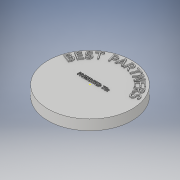
# Autodesk Inventor part: BEST PARTNERS
Saved by Autodesk Inventor 2018.2 (Build 222227000, 227)
## iProperties
Created: 2018-03-07
Part Number: BEST PARTNERS
Material: Generic
Document SubType Name: Modeling
Designer: battin.michael
Density: 1 g/cm^3
Appearance: Default
Author: battin.michael
Autodesk Inventor part; units mm, degrees
ref_plane "YZ Plane" through (0, 0, 0) normal (1, 0, 0) x (0, 1, 0)
ref_plane "XZ Plane" through (0, 0, 0) normal (0, 1, 0) x (-1, 0, 0)
ref_plane "XY Plane" through (0, 0, 0) normal (0, 0, 1) x (1, 0, 0)
sketch "Sketch1" plane through (0, 0, 0) normal (0, 1, 0) x (-1, 0, 0)
  circle A0 centre (0, 0) radius 104.775
  dimension "d0" = 209.55
  constraints: 1 centre point, 1 coincident
  measures "d0" diameter of A0
extrude "Extrusion1" add sketch "Sketch1" along normal blind 25.4
sketch "Sketch2" plane through (0, 25.4, 0) normal (0, 1, 0) x (1, 0, 0)
  circle A0 centre (0, 0) radius 104.775
  circle A1 centre (0, 0) radius 104.775 projected
  spline S0 degree 2 poles (-32.6567, 10.8601) (-32.6567, 10.3661) (-33.0087, 9.4769) (-33.3236, 9.1681) knots 0 0 0 1 2 2 2
  spline S1 degree 2 poles (-33.3236, 9.1681) (-33.7188, 8.7791) (-34.7871, 8.3777) (-35.6022, 8.3777) knots 0 0 0 1 2 2 2
  line L0 (-35.6022, 8.3777) -> (-36.4605, 8.3777)
  line L1 (-36.4605, 8.3777) -> (-36.4605, 5.5372)
  line L2 (-36.4605, 5.5372) -> (-37.4732, 5.5372)
  line L3 (-37.4732, 5.5372) -> (-37.4732, 13.1572)
  line L4 (-37.4732, 13.1572) -> (-35.559, 13.1572)
  spline S2 degree 2 poles (-35.559, 13.1572) (-34.8797, 13.1572) (-33.9288, 12.9349) (-33.5644, 12.6817) knots 0 0 0 1 2 2 2
  spline S3 degree 2 poles (-33.5644, 12.6817) (-33.1384, 12.3915) (-32.6567, 11.4961) (-32.6567, 10.8601) knots 0 0 0 1 2 2 2
  spline S4 degree 2 poles (-33.7126, 10.8292) (-33.7126, 11.2244) (-33.9843, 11.8049) (-34.2622, 11.9901) knots 0 0 0 1 2 2 2
  spline S5 degree 2 poles (-34.2622, 11.9901) (-34.503, 12.1507) (-35.1452, 12.2803) (-35.6207, 12.2803) knots 0 0 0 1 2 2 2
  line L5 (-35.6207, 12.2803) -> (-36.4605, 12.2803)
  line L6 (-36.4605, 12.2803) -> (-36.4605, 9.2422)
  line L7 (-36.4605, 9.2422) -> (-35.7689, 9.2422)
  spline S6 degree 2 poles (-35.7689, 9.2422) (-35.1514, 9.2422) (-34.3919, 9.4398) (-34.1449, 9.6992) knots 0 0 0 1 2 2 2
  spline S7 degree 2 poles (-34.1449, 9.6992) (-33.9164, 9.9277) (-33.7126, 10.4649) (-33.7126, 10.8292) knots 0 0 0 1 2 2 2
  line L8 (-25.7962, 5.5372) -> (-27.1115, 5.5372)
  line L9 (-27.1115, 5.5372) -> (-29.5198, 8.5691)
  line L10 (-29.5198, 8.5691) -> (-30.6807, 8.5691)
  line L11 (-30.6807, 8.5691) -> (-30.6807, 5.5372)
  line L12 (-30.6807, 5.5372) -> (-31.6934, 5.5372)
  line L13 (-31.6934, 5.5372) -> (-31.6934, 13.1572)
  line L14 (-31.6934, 13.1572) -> (-29.7297, 13.1572)
  spline S8 degree 2 poles (-29.7297, 13.1572) (-29.0752, 13.1572) (-28.1921, 13.0152) (-27.7908, 12.7558) knots 0 0 0 1 2 2 2
  spline S9 degree 2 poles (-27.7908, 12.7558) (-27.3894, 12.4965) (-26.9263, 11.6875) (-26.9263, 11.0886) knots 0 0 0 1 2 2 2
  spline S10 degree 2 poles (-26.9263, 11.0886) (-26.9263, 10.2549) (-27.7784, 9.1249) (-28.5071, 8.8532) knots 0 0 0 1 2 2 2
  line L15 (-28.5071, 8.8532) -> (-25.7962, 5.5372)
  spline S11 degree 2 poles (-27.9822, 11.0083) (-27.9822, 11.3417) (-28.2168, 11.8543) (-28.4638, 12.021) knots 0 0 0 1 2 2 2
  spline S12 degree 2 poles (-28.4638, 12.021) (-28.68, 12.163) (-29.2543, 12.2803) (-29.6742, 12.2803) knots 0 0 0 1 2 2 2
  line L16 (-29.6742, 12.2803) -> (-30.6807, 12.2803)
  line L17 (-30.6807, 12.2803) -> (-30.6807, 9.4151)
  line L18 (-30.6807, 9.4151) -> (-29.7915, 9.4151)
  spline S13 degree 2 poles (-29.7915, 9.4151) (-29.3531, 9.4151) (-28.6553, 9.5695) (-28.4144, 9.8103) knots 0 0 0 1 2 2 2
  spline S14 degree 2 poles (-28.4144, 9.8103) (-28.1921, 10.0203) (-27.9822, 10.6131) (-27.9822, 11.0083) knots 0 0 0 1 2 2 2
  line L19 (-25.1911, 5.5372) -> (-25.1911, 13.1572)
  line L20 (-25.1911, 13.1572) -> (-20.4239, 13.1572)
  line L21 (-20.4239, 13.1572) -> (-20.4239, 12.2556)
  line L22 (-20.4239, 12.2556) -> (-24.1784, 12.2556)
  line L23 (-24.1784, 12.2556) -> (-24.1784, 10.1685)
  line L24 (-24.1784, 10.1685) -> (-20.6771, 10.1685)
  line L25 (-20.6771, 10.1685) -> (-20.6771, 9.2669)
  line L26 (-20.6771, 9.2669) -> (-24.1784, 9.2669)
  line L27 (-24.1784, 9.2669) -> (-24.1784, 6.4388)
  line L28 (-24.1784, 6.4388) -> (-20.4239, 6.4388)
  line L29 (-20.4239, 6.4388) -> (-20.4239, 5.5372)
  line L30 (-20.4239, 5.5372) -> (-25.1911, 5.5372)
  spline S15 degree 2 poles (-17.1882, 5.4013) (-18.0157, 5.4013) (-19.1766, 5.7472) (-19.6891, 5.9942) knots 0 0 0 1 2 2 2
  line L31 (-19.6891, 5.9942) -> (-19.6891, 7.2662)
  line L32 (-19.6891, 7.2662) -> (-19.615, 7.2662)
  spline S16 degree 2 poles (-19.615, 7.2662) (-19.1148, 6.7969) (-17.849, 6.2782) (-17.2623, 6.2782) knots 0 0 0 1 2 2 2
  spline S17 degree 2 poles (-17.2623, 6.2782) (-16.4225, 6.2782) (-15.5642, 6.976) (-15.5642, 7.5503) knots 0 0 0 1 2 2 2
  spline S18 degree 2 poles (-15.5642, 7.5503) (-15.5642, 8.0072) (-16.015, 8.5753) (-16.5028, 8.7173) knots 0 0 0 1 2 2 2
  spline S19 degree 2 poles (-16.5028, 8.7173) (-16.8548, 8.8161) (-17.4414, 8.952) (-17.8798, 9.0631) knots 0 0 0 1 2 2 2
  spline S20 degree 2 poles (-17.8798, 9.0631) (-18.275, 9.1681) (-18.8987, 9.4831) (-19.1395, 9.7362) knots 0 0 0 1 2 2 2
  spline S21 degree 2 poles (-19.1395, 9.7362) (-19.3742, 9.9894) (-19.6335, 10.6687) (-19.6335, 11.1133) knots 0 0 0 1 2 2 2
  spline S22 degree 2 poles (-19.6335, 11.1133) (-19.6335, 12.0395) (-18.1886, 13.2931) (-17.0709, 13.2931) knots 0 0 0 1 2 2 2
  spline S23 degree 2 poles (-17.0709, 13.2931) (-16.4287, 13.2931) (-15.2925, 13.0399) (-14.8047, 12.799) knots 0 0 0 1 2 2 2
  line L33 (-14.8047, 12.799) -> (-14.8047, 11.5887)
  line L34 (-14.8047, 11.5887) -> (-14.8788, 11.5887)
  spline S24 degree 2 poles (-14.8788, 11.5887) (-15.2431, 11.9222) (-16.3793, 12.4162) (-17.003, 12.4162) knots 0 0 0 1 2 2 2
  spline S25 degree 2 poles (-17.003, 12.4162) (-17.7069, 12.4162) (-18.5776, 11.7555) (-18.5776, 11.2182) knots 0 0 0 1 2 2 2
  spline S26 degree 2 poles (-18.5776, 11.2182) (-18.5776, 10.7366) (-18.0651, 10.1623) (-17.5834, 10.0326) knots 0 0 0 1 2 2 2
  spline S27 degree 2 poles (-17.5834, 10.0326) (-17.2623, 9.9462) (-16.3299, 9.7239) (-16.0211, 9.6313) knots 0 0 0 1 2 2 2
  spline S28 degree 2 poles (-16.0211, 9.6313) (-15.2369, 9.3904) (-14.5083, 8.4209) (-14.5083, 7.7108) knots 0 0 0 1 2 2 2
  spline S29 degree 2 poles (-14.5083, 7.7108) (-14.5083, 7.26) (-14.8726, 6.3955) (-15.1999, 6.093) knots 0 0 0 1 2 2 2
  spline S30 degree 2 poles (-15.1999, 6.093) (-15.5642, 5.7595) (-16.4904, 5.4013) (-17.1882, 5.4013) knots 0 0 0 1 2 2 2
  line L35 (-13.477, 5.5372) -> (-13.477, 13.1572)
  line L36 (-13.477, 13.1572) -> (-8.7099, 13.1572)
  line L37 (-8.7099, 13.1572) -> (-8.7099, 12.2556)
  line L38 (-8.7099, 12.2556) -> (-12.4643, 12.2556)
  line L39 (-12.4643, 12.2556) -> (-12.4643, 10.1685)
  line L40 (-12.4643, 10.1685) -> (-8.9631, 10.1685)
  line L41 (-8.9631, 10.1685) -> (-8.9631, 9.2669)
  line L42 (-8.9631, 9.2669) -> (-12.4643, 9.2669)
  line L43 (-12.4643, 9.2669) -> (-12.4643, 6.4388)
  line L44 (-12.4643, 6.4388) -> (-8.7099, 6.4388)
  line L45 (-8.7099, 6.4388) -> (-8.7099, 5.5372)
  line L46 (-8.7099, 5.5372) -> (-13.477, 5.5372)
  line L47 (-2.1458, 5.5372) -> (-3.282, 5.5372)
  line L48 (-3.282, 5.5372) -> (-6.6536, 12.1074)
  line L49 (-6.6536, 12.1074) -> (-6.6536, 5.5372)
  line L50 (-6.6536, 5.5372) -> (-7.5984, 5.5372)
  line L51 (-7.5984, 5.5372) -> (-7.5984, 13.1572)
  line L52 (-7.5984, 13.1572) -> (-6.1596, 13.1572)
  line L53 (-6.1596, 13.1572) -> (-3.0906, 7.1242)
  line L54 (-3.0906, 7.1242) -> (-3.0906, 13.1572)
  line L55 (-3.0906, 13.1572) -> (-2.1458, 13.1572)
  line L56 (-2.1458, 13.1572) -> (-2.1458, 5.5372)
  line L57 (1.1763, 5.5372) -> (1.1763, 12.2556)
  line L58 (1.1763, 12.2556) -> (-1.3801, 12.2556)
  line L59 (-1.3801, 12.2556) -> (-1.3801, 13.1572)
  line L60 (-1.3801, 13.1572) -> (4.7455, 13.1572)
  line L61 (4.7455, 13.1572) -> (4.7455, 12.2556)
  line L62 (4.7455, 12.2556) -> (2.1891, 12.2556)
  line L63 (2.1891, 12.2556) -> (2.1891, 5.5372)
  line L64 (2.1891, 5.5372) -> (1.1763, 5.5372)
  line L65 (5.5174, 5.5372) -> (5.5174, 13.1572)
  line L66 (5.5174, 13.1572) -> (10.2845, 13.1572)
  line L67 (10.2845, 13.1572) -> (10.2845, 12.2556)
  line L68 (10.2845, 12.2556) -> (6.5301, 12.2556)
  line L69 (6.5301, 12.2556) -> (6.5301, 10.1685)
  line L70 (6.5301, 10.1685) -> (10.0314, 10.1685)
  line L71 (10.0314, 10.1685) -> (10.0314, 9.2669)
  line L72 (10.0314, 9.2669) -> (6.5301, 9.2669)
  line L73 (6.5301, 9.2669) -> (6.5301, 6.4388)
  line L74 (6.5301, 6.4388) -> (10.2845, 6.4388)
  line L75 (10.2845, 6.4388) -> (10.2845, 5.5372)
  line L76 (10.2845, 5.5372) -> (5.5174, 5.5372)
  spline S31 degree 2 poles (17.4044, 9.341) (17.4044, 8.2974) (16.5584, 6.6178) (15.8482, 6.1485) knots 0 0 0 1 2 2 2
  spline S32 degree 2 poles (15.8482, 6.1485) (15.2678, 5.7842) (14.076, 5.5372) (13.1498, 5.5372) knots 0 0 0 1 2 2 2
  line L77 (13.1498, 5.5372) -> (11.396, 5.5372)
  line L78 (11.396, 5.5372) -> (11.396, 13.1572)
  line L79 (11.396, 13.1572) -> (13.1312, 13.1572)
  spline S33 degree 2 poles (13.1312, 13.1572) (14.2057, 13.1572) (15.4283, 12.8361) (15.8606, 12.552) knots 0 0 0 1 2 2 2
  spline S34 degree 2 poles (15.8606, 12.552) (16.5954, 12.0642) (17.4044, 10.4525) (17.4044, 9.341) knots 0 0 0 1 2 2 2
  spline S35 degree 2 poles (16.3484, 9.3534) (16.3484, 10.2302) (15.768, 11.4714) (15.1937, 11.8234) knots 0 0 0 1 2 2 2
  spline S36 degree 2 poles (15.1937, 11.8234) (14.7861, 12.0642) (13.8661, 12.2803) (13.1806, 12.2803) knots 0 0 0 1 2 2 2
  line L80 (13.1806, 12.2803) -> (12.4087, 12.2803)
  line L81 (12.4087, 12.2803) -> (12.4087, 6.4141)
  line L82 (12.4087, 6.4141) -> (13.1806, 6.4141)
  spline S37 degree 2 poles (13.1806, 6.4141) (13.8537, 6.4141) (14.8726, 6.6302) (15.2863, 6.9204) knots 0 0 0 1 2 2 2
  spline S38 degree 2 poles (15.2863, 6.9204) (15.8174, 7.2786) (16.3484, 8.4642) (16.3484, 9.3534) knots 0 0 0 1 2 2 2
  line L83 (23.5547, 5.5372) -> (23.5547, 12.2556)
  line L84 (23.5547, 12.2556) -> (20.9982, 12.2556)
  line L85 (20.9982, 12.2556) -> (20.9982, 13.1572)
  line L86 (20.9982, 13.1572) -> (27.1239, 13.1572)
  line L87 (27.1239, 13.1572) -> (27.1239, 12.2556)
  line L88 (27.1239, 12.2556) -> (24.5674, 12.2556)
  line L89 (24.5674, 12.2556) -> (24.5674, 5.5372)
  line L90 (24.5674, 5.5372) -> (23.5547, 5.5372)
  spline S39 degree 2 poles (33.2866, 12.2865) (33.7188, 11.7802) (34.2005, 10.2982) (34.2005, 9.3472) knots 0 0 0 1 2 2 2
  spline S40 degree 2 poles (34.2005, 9.3472) (34.2005, 8.4209) (33.7312, 6.9204) (33.2866, 6.4141) knots 0 0 0 1 2 2 2
  spline S41 degree 2 poles (33.2866, 6.4141) (32.8173, 5.883) (31.5761, 5.3766) (30.8289, 5.3766) knots 0 0 0 1 2 2 2
  spline S42 degree 2 poles (30.8289, 5.3766) (30.057, 5.3766) (28.822, 5.9015) (28.3712, 6.4141) knots 0 0 0 1 2 2 2
  spline S43 degree 2 poles (28.3712, 6.4141) (27.9328, 6.9204) (27.4635, 8.4086) (27.4635, 9.3472) knots 0 0 0 1 2 2 2
  spline S44 degree 2 poles (27.4635, 9.3472) (27.4635, 10.3043) (27.939, 11.7616) (28.3774, 12.2865) knots 0 0 0 1 2 2 2
  spline S45 degree 2 poles (28.3774, 12.2865) (28.822, 12.7929) (30.0632, 13.3178) (30.8289, 13.3178) knots 0 0 0 1 2 2 2
  spline S46 degree 2 poles (30.8289, 13.3178) (31.6069, 13.3178) (32.8543, 12.7743) (33.2866, 12.2865) knots 0 0 0 1 2 2 2
  spline S47 degree 2 poles (33.1445, 9.3472) (33.1445, 10.1006) (32.8173, 11.2676) (32.5209, 11.6505) knots 0 0 0 1 2 2 2
  spline S48 degree 2 poles (32.5209, 11.6505) (32.2183, 12.0457) (31.3661, 12.4409) (30.8351, 12.4409) knots 0 0 0 1 2 2 2
  spline S49 degree 2 poles (30.8351, 12.4409) (30.2855, 12.4409) (29.458, 12.058) (29.1431, 11.6505) knots 0 0 0 1 2 2 2
  spline S50 degree 2 poles (29.1431, 11.6505) (28.8405, 11.2615) (28.5194, 10.0882) (28.5194, 9.3472) knots 0 0 0 1 2 2 2
  spline S51 degree 2 poles (28.5194, 9.3472) (28.5194, 7.8467) (29.7791, 6.2535) (30.8351, 6.2535) knots 0 0 0 1 2 2 2
  spline S52 degree 2 poles (30.8351, 6.2535) (31.891, 6.2535) (33.1445, 7.8467) (33.1445, 9.3472) knots 0 0 0 1 2 2 2
  line L91 (37.0039, 5.5372) -> (35.7813, 5.5372)
  line L92 (35.7813, 5.5372) -> (35.7813, 6.9945)
  line L93 (35.7813, 6.9945) -> (37.0039, 6.9945)
  line L94 (37.0039, 6.9945) -> (37.0039, 5.5372)
  line L95 (37.0039, 9.798) -> (35.7813, 9.798)
  line L96 (35.7813, 9.798) -> (35.7813, 11.2553)
  line L97 (35.7813, 11.2553) -> (37.0039, 11.2553)
  line L98 (37.0039, 11.2553) -> (37.0039, 9.798)
  spline S53 degree 2 poles (-76.2187, 36.9163) (-74.8015, 36.3811) (-73.0366, 34.4825) (-72.6654, 33.3214) knots 0 0 0 1 2 2 2
  spline S54 degree 2 poles (-72.6654, 33.3214) (-72.2408, 31.9289) (-72.4572, 29.2119) (-73.1902, 27.2709) knots 0 0 0 1 2 2 2
  line L99 (-73.1902, 27.2709) -> (-75.2497, 21.8176)
  line L100 (-75.2497, 21.8176) -> (-94.2593, 28.9966)
  line L101 (-94.2593, 28.9966) -> (-92.3569, 34.034)
  spline S55 degree 2 poles (-92.3569, 34.034) (-91.5889, 36.0674) (-90.5591, 38.002) (-89.7017, 38.7343) knots 0 0 0 1 2 2 2
  spline S56 degree 2 poles (-89.7017, 38.7343) (-88.7728, 39.5628) (-86.6463, 39.8334) (-85.4447, 39.3796) knots 0 0 0 1 2 2 2
  spline S57 degree 2 poles (-85.4447, 39.3796) (-84.1045, 38.8735) (-82.5139, 36.6534) (-82.3843, 35.1787) knots 0 0 0 1 2 2 2
  line L102 (-82.3843, 35.1787) -> (-82.2919, 35.1438)
  spline S58 degree 2 poles (-82.2919, 35.1438) (-81.1898, 36.6638) (-78.0365, 37.6028) (-76.2187, 36.9163) knots 0 0 0 1 2 2 2
  spline S59 degree 2 poles (-77.1057, 34.2414) (-78.1841, 34.6486) (-79.8032, 34.556) (-80.6452, 33.8179) knots 0 0 0 1 2 2 2
  spline S60 degree 2 poles (-80.6452, 33.8179) (-81.1802, 33.3334) (-81.9003, 31.986) (-82.3948, 30.6766) knots 0 0 0 1 2 2 2
  line L103 (-82.3948, 30.6766) -> (-83.4769, 27.8113)
  line L104 (-83.4769, 27.8113) -> (-76.4523, 25.1584)
  line L105 (-76.4523, 25.1584) -> (-75.6785, 27.2073)
  spline S61 degree 2 poles (-75.6785, 27.2073) (-75.0502, 28.871) (-74.6369, 30.8976) (-74.8506, 31.8232) knots 0 0 0 1 2 2 2
  spline S62 degree 2 poles (-74.8506, 31.8232) (-75.0914, 32.7238) (-76.1044, 33.8632) (-77.1057, 34.2414) knots 0 0 0 1 2 2 2
  spline S63 degree 2 poles (-86.0853, 36.6116) (-86.7631, 36.8676) (-87.9543, 36.7894) (-88.439, 36.3916) knots 0 0 0 1 2 2 2
  spline S64 degree 2 poles (-88.439, 36.3916) (-89.0106, 35.9034) (-89.729, 34.4673) (-90.2351, 33.1271) knots 0 0 0 1 2 2 2
  line L106 (-90.2351, 33.1271) -> (-91.1485, 30.7085)
  line L107 (-91.1485, 30.7085) -> (-85.5873, 28.6083)
  line L108 (-85.5873, 28.6083) -> (-84.5053, 31.4736)
  spline S65 degree 2 poles (-84.5053, 31.4736) (-84.0573, 32.6598) (-83.8791, 33.8774) (-84.0373, 34.6237) knots 0 0 0 1 2 2 2
  spline S66 degree 2 poles (-84.0373, 34.6237) (-84.1859, 35.3487) (-85.1918, 36.2742) (-86.0853, 36.6116) knots 0 0 0 1 2 2 2
  line L109 (-69.019, 37.0158) -> (-86.1686, 47.915)
  line L110 (-86.1686, 47.915) -> (-79.35, 58.644)
  line L111 (-79.35, 58.644) -> (-77.321, 57.3544)
  line L112 (-77.321, 57.3544) -> (-82.6911, 48.9047)
  line L113 (-82.6911, 48.9047) -> (-77.9937, 45.9194)
  line L114 (-77.9937, 45.9194) -> (-72.9857, 53.7993)
  line L115 (-72.9857, 53.7993) -> (-70.9567, 52.5097)
  line L116 (-70.9567, 52.5097) -> (-75.9647, 44.6298)
  line L117 (-75.9647, 44.6298) -> (-69.5996, 40.5846)
  line L118 (-69.5996, 40.5846) -> (-64.2294, 49.0343)
  line L119 (-64.2294, 49.0343) -> (-62.2004, 47.7448)
  line L120 (-62.2004, 47.7448) -> (-69.019, 37.0158)
  spline S67 degree 2 poles (-56.098, 53.8234) (-57.6268, 52.2323) (-60.4367, 50.6389) (-61.8586, 50.1098) knots 0 0 0 1 2 2 2
  line L121 (-61.8586, 50.1098) -> (-64.3046, 52.4601)
  line L122 (-64.3046, 52.4601) -> (-64.1676, 52.6026)
  spline S68 degree 2 poles (-64.1676, 52.6026) (-62.3411, 52.6972) (-59.0048, 54.173) (-57.9209, 55.301) knots 0 0 0 1 2 2 2
  spline S69 degree 2 poles (-57.9209, 55.301) (-56.3693, 56.9158) (-56.1252, 59.8555) (-57.2294, 60.9165) knots 0 0 0 1 2 2 2
  spline S70 degree 2 poles (-57.2294, 60.9165) (-58.1081, 61.7608) (-60.0333, 61.9437) (-61.2077, 61.2681) knots 0 0 0 1 2 2 2
  spline S71 degree 2 poles (-61.2077, 61.2681) (-62.048, 60.7738) (-63.3931, 59.8968) (-64.4169, 59.2591) knots 0 0 0 1 2 2 2
  spline S72 degree 2 poles (-64.4169, 59.2591) (-65.349, 58.6932) (-67.1068, 58.0758) (-68.0386, 58.0805) knots 0 0 0 1 2 2 2
  spline S73 degree 2 poles (-68.0386, 58.0805) (-68.959, 58.0971) (-70.7443, 58.8534) (-71.5992, 59.6749) knots 0 0 0 1 2 2 2
  spline S74 degree 2 poles (-71.5992, 59.6749) (-73.3803, 61.3862) (-73.1209, 66.4808) (-71.0558, 68.6299) knots 0 0 0 1 2 2 2
  spline S75 degree 2 poles (-71.0558, 68.6299) (-69.8692, 69.8648) (-67.2831, 71.5817) (-65.9187, 72.0748) knots 0 0 0 1 2 2 2
  line L123 (-65.9187, 72.0748) -> (-63.5915, 69.8386)
  line L124 (-63.5915, 69.8386) -> (-63.7284, 69.6961)
  spline S76 degree 2 poles (-63.7284, 69.6961) (-65.0427, 69.6117) (-68.0919, 68.3396) (-69.2442, 67.1404) knots 0 0 0 1 2 2 2
  spline S77 degree 2 poles (-69.2442, 67.1404) (-70.5449, 65.7868) (-70.8831, 62.8918) (-69.8501, 61.8992) knots 0 0 0 1 2 2 2
  spline S78 degree 2 poles (-69.8501, 61.8992) (-68.9239, 61.0093) (-66.8727, 60.9338) (-65.7334, 61.6203) knots 0 0 0 1 2 2 2
  spline S79 degree 2 poles (-65.7334, 61.6203) (-64.9739, 62.078) (-62.8237, 63.4602) (-62.0751, 63.8828) knots 0 0 0 1 2 2 2
  spline S80 degree 2 poles (-62.0751, 63.8828) (-60.1631, 64.9458) (-56.9526, 64.5556) (-55.5872, 63.2436) knots 0 0 0 1 2 2 2
  spline S81 degree 2 poles (-55.5872, 63.2436) (-54.7204, 62.4107) (-53.7312, 60.1129) (-53.7541, 58.9245) knots 0 0 0 1 2 2 2
  spline S82 degree 2 poles (-53.7541, 58.9245) (-53.786, 57.6079) (-54.8087, 55.1651) (-56.098, 53.8234) knots 0 0 0 1 2 2 2
  line L125 (-45.3482, 63.6066) -> (-55.4918, 78.3743)
  line L126 (-55.4918, 78.3743) -> (-61.1111, 74.5145)
  line L127 (-61.1111, 74.5145) -> (-62.4723, 76.4962)
  line L128 (-62.4723, 76.4962) -> (-49.0076, 85.7448)
  line L129 (-49.0076, 85.7448) -> (-47.6465, 83.7631)
  line L130 (-47.6465, 83.7631) -> (-53.2658, 79.9033)
  line L131 (-53.2658, 79.9033) -> (-43.1222, 65.1356)
  line L132 (-43.1222, 65.1356) -> (-45.3482, 63.6066)
  spline S83 degree 2 poles (-19.2896, 90.5476) (-18.9158, 89.2844) (-19.143, 86.7443) (-19.7146, 85.7165) knots 0 0 0 1 2 2 2
  spline S84 degree 2 poles (-19.7146, 85.7165) (-20.4308, 84.4227) (-22.8588, 82.588) (-24.9431, 81.9713) knots 0 0 0 1 2 2 2
  line L133 (-24.9431, 81.9713) -> (-27.1379, 81.3218)
  line L134 (-27.1379, 81.3218) -> (-24.9886, 74.0584)
  line L135 (-24.9886, 74.0584) -> (-27.5781, 73.2922)
  line L136 (-27.5781, 73.2922) -> (-33.3439, 92.777)
  line L137 (-33.3439, 92.777) -> (-28.449, 94.2254)
  spline S85 degree 2 poles (-28.449, 94.2254) (-26.7121, 94.7394) (-24.1122, 94.8905) (-22.989, 94.5188) knots 0 0 0 1 2 2 2
  spline S86 degree 2 poles (-22.989, 94.5188) (-21.6799, 94.0991) (-19.7708, 92.174) (-19.2896, 90.5476) knots 0 0 0 1 2 2 2
  spline S87 degree 2 poles (-21.9663, 89.6697) (-22.2653, 90.6802) (-23.3993, 91.9589) (-24.25, 92.2223) knots 0 0 0 1 2 2 2
  spline S88 degree 2 poles (-24.25, 92.2223) (-24.9873, 92.4506) (-26.7276, 92.2963) (-27.9434, 91.9365) knots 0 0 0 1 2 2 2
  line L138 (-27.9434, 91.9365) -> (-30.0908, 91.3011)
  line L139 (-30.0908, 91.3011) -> (-27.792, 83.5324)
  line L140 (-27.792, 83.5324) -> (-26.0235, 84.0557)
  spline S89 degree 2 poles (-26.0235, 84.0557) (-24.4445, 84.523) (-22.6519, 85.603) (-22.2165, 86.453) knots 0 0 0 1 2 2 2
  spline S90 degree 2 poles (-22.2165, 86.453) (-21.8052, 87.2101) (-21.6906, 88.7381) (-21.9663, 89.6697) knots 0 0 0 1 2 2 2
  line L141 (-14.9194, 77.1527) -> (-9.7313, 97.9592)
  line L142 (-9.7313, 97.9592) -> (-6.4158, 98.2276)
  line L143 (-6.4158, 98.2276) -> (2.0517, 78.5266)
  line L144 (2.0517, 78.5266) -> (-0.7878, 78.2968)
  line L145 (-0.7878, 78.2968) -> (-3.0845, 83.8105)
  line L146 (-3.0845, 83.8105) -> (-10.815, 83.1846)
  line L147 (-10.815, 83.1846) -> (-12.1949, 77.3733)
  line L148 (-12.1949, 77.3733) -> (-14.9194, 77.1527)
  line L149 (-4.0091, 86.0485) -> (-7.916, 95.3307)
  line L150 (-7.916, 95.3307) -> (-10.2625, 85.5422)
  line L151 (-10.2625, 85.5422) -> (-4.0091, 86.0485)
  line L152 (19.7977, 76.102) -> (16.3238, 76.5857)
  line L153 (16.3238, 76.5857) -> (11.078, 85.4792)
  line L154 (11.078, 85.4792) -> (8.0118, 85.9061)
  line L155 (8.0118, 85.9061) -> (6.8969, 77.8981)
  line L156 (6.8969, 77.8981) -> (4.2222, 78.2705)
  line L157 (4.2222, 78.2705) -> (7.0242, 98.3964)
  line L158 (7.0242, 98.3964) -> (12.2106, 97.6743)
  spline S91 degree 2 poles (12.2106, 97.6743) (13.9394, 97.4336) (16.2194, 96.7338) (17.1842, 95.9012) knots 0 0 0 1 2 2 2
  spline S92 degree 2 poles (17.1842, 95.9012) (18.1489, 95.0686) (19.0747, 92.7618) (18.8544, 91.1797) knots 0 0 0 1 2 2 2
  spline S93 degree 2 poles (18.8544, 91.1797) (18.5479, 88.978) (15.8816, 86.3067) (13.8572, 85.857) knots 0 0 0 1 2 2 2
  line L159 (13.8572, 85.857) -> (19.7977, 76.102)
  spline S94 degree 2 poles (16.036, 91.356) (16.1586, 92.2367) (15.7273, 93.6767) (15.1362, 94.2079) knots 0 0 0 1 2 2 2
  spline S95 degree 2 poles (15.1362, 94.2079) (14.6176, 94.6625) (13.144, 95.1835) (12.035, 95.3379) knots 0 0 0 1 2 2 2
  line L160 (12.035, 95.3379) -> (9.3765, 95.7081)
  line L161 (9.3765, 95.7081) -> (8.3229, 88.1405)
  line L162 (8.3229, 88.1405) -> (10.6715, 87.8135)
  spline S96 degree 2 poles (10.6715, 87.8135) (11.8294, 87.6523) (13.7292, 87.8034) (14.4538, 88.3509) knots 0 0 0 1 2 2 2
  spline S97 degree 2 poles (14.4538, 88.3509) (15.1182, 88.8237) (15.8907, 90.3122) (16.036, 91.356) knots 0 0 0 1 2 2 2
  line L163 (25.7253, 73.7595) -> (31.9204, 90.5702)
  line L164 (31.9204, 90.5702) -> (25.5237, 92.9275)
  line L165 (25.5237, 92.9275) -> (26.355, 95.1834)
  line L166 (26.355, 95.1834) -> (41.6824, 89.5349)
  line L167 (41.6824, 89.5349) -> (40.8511, 87.279)
  line L168 (40.8511, 87.279) -> (34.4544, 89.6364)
  line L169 (34.4544, 89.6364) -> (28.2593, 72.8257)
  line L170 (28.2593, 72.8257) -> (25.7253, 73.7595)
  line L171 (48.6475, 61.5359) -> (46.1067, 63.1865)
  line L172 (46.1067, 63.1865) -> (48.1124, 82.777)
  line L173 (48.1124, 82.777) -> (38.5673, 68.0847)
  line L174 (38.5673, 68.0847) -> (36.4546, 69.4572)
  line L175 (36.4546, 69.4572) -> (47.5248, 86.497)
  line L176 (47.5248, 86.497) -> (50.7422, 84.4068)
  line L177 (50.7422, 84.4068) -> (48.8404, 66.4572)
  line L178 (48.8404, 66.4572) -> (57.605, 79.9482)
  line L179 (57.605, 79.9482) -> (59.7177, 78.5756)
  line L180 (59.7177, 78.5756) -> (48.6475, 61.5359)
  line L181 (51.7107, 58.8201) -> (66.2169, 73.0494)
  line L182 (66.2169, 73.0494) -> (75.1189, 63.9742)
  line L183 (75.1189, 63.9742) -> (73.4026, 62.2906)
  line L184 (73.4026, 62.2906) -> (66.3917, 69.4379)
  line L185 (66.3917, 69.4379) -> (62.4184, 65.5404)
  line L186 (62.4184, 65.5404) -> (68.9565, 58.8751)
  line L187 (68.9565, 58.8751) -> (67.2402, 57.1916)
  line L188 (67.2402, 57.1916) -> (60.7021, 63.8569)
  line L189 (60.7021, 63.8569) -> (55.3181, 58.5757)
  line L190 (55.3181, 58.5757) -> (62.329, 51.4284)
  line L191 (62.329, 51.4284) -> (60.6127, 49.7449)
  line L192 (60.6127, 49.7449) -> (51.7107, 58.8201)
  line L193 (70.8399, 34.1346) -> (68.9614, 37.0965)
  line L194 (68.9614, 37.0965) -> (72.3497, 46.8501)
  line L195 (72.3497, 46.8501) -> (70.6917, 49.4644)
  line L196 (70.6917, 49.4644) -> (63.8639, 45.1342)
  line L197 (63.8639, 45.1342) -> (62.4175, 47.4147)
  line L198 (62.4175, 47.4147) -> (79.5774, 58.2977)
  line L199 (79.5774, 58.2977) -> (82.3819, 53.8757)
  spline S98 degree 2 poles (82.3819, 53.8757) (83.3168, 52.4016) (84.2581, 50.2102) (84.2473, 48.9359) knots 0 0 0 1 2 2 2
  spline S99 degree 2 poles (84.2473, 48.9359) (84.2365, 47.6616) (83.0763, 45.4634) (81.7274, 44.6079) knots 0 0 0 1 2 2 2
  spline S100 degree 2 poles (81.7274, 44.6079) (79.8501, 43.4173) (76.0883, 43.7224) (74.4357, 44.9752) knots 0 0 0 1 2 2 2
  line L200 (74.4357, 44.9752) -> (70.8399, 34.1346)
  spline S101 degree 2 poles (80.0385, 46.8712) (80.7895, 47.3474) (81.6085, 48.6078) (81.6312, 49.4022) knots 0 0 0 1 2 2 2
  spline S102 degree 2 poles (81.6312, 49.4022) (81.6424, 50.0917) (81.0864, 51.5526) (80.4867, 52.4982) knots 0 0 0 1 2 2 2
  line L201 (80.4867, 52.4982) -> (79.0491, 54.7648)
  line L202 (79.0491, 54.7648) -> (72.5968, 50.6727)
  line L203 (72.5968, 50.6727) -> (73.8668, 48.6702)
  spline S103 degree 2 poles (73.8668, 48.6702) (74.4929, 47.6829) (75.8372, 46.332) (76.7234, 46.1336) knots 0 0 0 1 2 2 2
  spline S104 degree 2 poles (76.7234, 46.1336) (77.5137, 45.9329) (79.1486, 46.3067) (80.0385, 46.8712) knots 0 0 0 1 2 2 2
  spline S105 degree 2 poles (72.8655, 27.1027) (72.0978, 29.1714) (71.8852, 32.3946) (72.0272, 33.9051) knots 0 0 0 1 2 2 2
  line L204 (72.0272, 33.9051) -> (75.2074, 35.0853)
  line L205 (75.2074, 35.0853) -> (75.2762, 34.9)
  spline S106 degree 2 poles (75.2762, 34.9) (74.567, 33.2141) (74.4447, 29.5681) (74.9889, 28.1015) knots 0 0 0 1 2 2 2
  spline S107 degree 2 poles (74.9889, 28.1015) (75.7681, 26.0019) (78.309, 24.5035) (79.7447, 25.0363) knots 0 0 0 1 2 2 2
  spline S108 degree 2 poles (79.7447, 25.0363) (80.8871, 25.4602) (81.8892, 27.1143) (81.7916, 28.4657) knots 0 0 0 1 2 2 2
  spline S109 degree 2 poles (81.7916, 28.4657) (81.7121, 29.4373) (81.5074, 31.0299) (81.3785, 32.2292) knots 0 0 0 1 2 2 2
  spline S110 degree 2 poles (81.3785, 32.2292) (81.2743, 33.3146) (81.483, 35.166) (81.8925, 36.003) knots 0 0 0 1 2 2 2
  spline S111 degree 2 poles (81.8925, 36.003) (82.3078, 36.8245) (83.7653, 38.1031) (84.8768, 38.5156) knots 0 0 0 1 2 2 2
  spline S112 degree 2 poles (84.8768, 38.5156) (87.1925, 39.375) (91.6671, 36.9256) (92.7041, 34.1313) knots 0 0 0 1 2 2 2
  spline S113 degree 2 poles (92.7041, 34.1313) (93.2999, 32.5258) (93.7211, 29.4503) (93.5716, 28.0072) knots 0 0 0 1 2 2 2
  line L206 (93.5716, 28.0072) -> (90.5458, 26.8843)
  line L207 (90.5458, 26.8843) -> (90.4771, 27.0696)
  spline S114 degree 2 poles (90.4771, 27.0696) (90.9727, 28.2898) (91.1535, 31.5887) (90.5749, 33.1479) knots 0 0 0 1 2 2 2
  spline S115 degree 2 poles (90.5749, 33.1479) (89.9218, 34.9079) (87.4621, 36.4716) (86.119, 35.9732) knots 0 0 0 1 2 2 2
  spline S116 degree 2 poles (86.119, 35.9732) (84.9148, 35.5263) (83.9546, 33.7121) (84.0773, 32.3876) knots 0 0 0 1 2 2 2
  spline S117 degree 2 poles (84.0773, 32.3876) (84.1591, 31.5046) (84.4684, 28.9673) (84.5233, 28.1094) knots 0 0 0 1 2 2 2
  spline S118 degree 2 poles (84.5233, 28.1094) (84.6488, 25.9254) (82.9011, 23.2042) (81.1258, 22.5453) knots 0 0 0 1 2 2 2
  spline S119 degree 2 poles (81.1258, 22.5453) (79.9988, 22.1271) (77.4995, 22.2359) (76.4393, 22.7733) knots 0 0 0 1 2 2 2
  spline S120 degree 2 poles (76.4393, 22.7733) (75.2677, 23.3748) (73.5129, 25.3582) (72.8655, 27.1027) knots 0 0 0 1 2 2 2
  point P0 (-38.2451, 5.5372)
  constraints: 1 centre point, 1 coincident, 2 other
extrude "Extrusion2" add sketch "Sketch2" along normal blind 2.54 contours S0 S1 L0 L1 L2 L3 L4 S2 S3 | L8 L9 L10 L11 L12 L13 L14 S8 S9 S10 L15 | L19 L20 L21 L22 L23 L24 L25 L26 L27 L28 L29 L30 | S15 L31 L32 S16 S17 S18 S19 S20 S21 S22 S23 L33 L34 S24 S25 S26 S27 S28 S29 S30 | L35 L36 L37 L38 L39 L40 L41 L42 L43 L44 L45 L46 | L47 L48 L49 L50 L51 L52 L53 L54 L55 L56 | L57 L58 L59 L60 L61 L62 L63 L64 | L65 L66 L67 L68 L69 L70 L71 L72 L73 L74 L75 L76 | S31 S32 L77 L78 L79 S33 S34 | L83 L84 L85 L86 L87 L88 L89 L90 | S39 S40 S41 S42 S43 S44 S45 S46 | L91 L92 L93 L94 | L95 L96 L97 L98 | S53 S54 L99 L100 L101 S55 S56 S57 L102 S58 | L109 L110 L111 L112 L113 L114 L115 L116 L117 L118 L119 L120 | S67 L121 L122 S68 S69 S70 S71 S72 S73 S74 S75 L123 L124 S76 S77 S78 S79 S80 S81 S82 | L125 L126 L127 L128 L129 L130 L131 L132 | S83 S84 L133 L134 L135 L136 L137 S85 S86 | L141 L142 L143 L144 L145 L146 L147 L148 | L152 L153 L154 L155 L156 L157 L158 S91 S92 S93 L159 | L163 L164 L165 L166 L167 L168 L169 L170 | L171 L172 L173 L174 L175 L176 L177 L178 L179 L180 | L181 L182 L183 L184 L185 L186 L187 L188 L189 L190 L191 L192 | L193 L194 L195 L196 L197 L198 L199 S98 S99 S100 L200 | S105 L204 L205 S106 S107 S108 S109 S110 S111 S112 S113 L206 L207 S114 S115 S116 S117 S118 S119 S120
sketch "Sketch3" plane through (0, 25.4, 0) normal (0, 1, 0) x (1, 0, 0)
  point P0 (0, 0)
body "Solid1"
